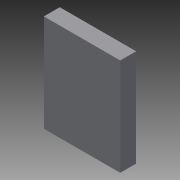
# Autodesk Inventor part: udoo
Saved by Autodesk Inventor 2015 (Build 190159000, 159)
## iProperties
Created: 2014-09-20
Part Number: udoo
Material: Generic
Document SubType Name: Modeling
Designer: ericd_000
Density: 1 g/cm^3
Appearance: Default
Author: ericd_000
Autodesk Inventor part; units mm, degrees
ref_plane "YZ Plane" through (0, 0, 0) normal (1, 0, 0) x (0, 1, 0)
ref_plane "XZ Plane" through (0, 0, 0) normal (0, 1, 0) x (-1, 0, 0)
ref_plane "XY Plane" through (0, 0, 0) normal (0, 0, 1) x (1, 0, 0)
sketch "Sketch1" plane through (0, 0, 0) normal (0, 1, 0) x (-1, 0, 0)
  line L0 (34.8904, 52.3767) -> (-51.4696, 52.3767)
  line L1 (-51.4696, 52.3767) -> (-51.4696, -57.6307)
  line L2 (-51.4696, -57.6307) -> (34.8904, -57.6307)
  line L3 (34.8904, -57.6307) -> (34.8904, 52.3767)
  point P0 (0, 0)
  dimension "d0" = 110.0074
  dimension "d1" = 86.36
  constraints: 8 end point, 2 parallel, 1 horizontal, 1 perpendicular
  measures "d0" distance of L2.end L0.start
  measures "d1" distance of L0.start L0.end
extrude "Extrusion1" add sketch "Sketch1" along normal blind 18
body "Solid1"
